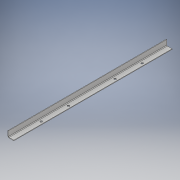
# Autodesk Inventor part: L_Profile
Saved by Autodesk Inventor 2019.3 (Build 233278000, 278)
## iProperties
Created: 2019-01-16
Part Number: L_Profile
Material: Generisch
Document SubType Name: Blech
Designer: Jonas
Density: 1 g/cm^3
Sheet Metal Rule: Standard_mm
Appearance: Vorgabe
Author: Jonas
Autodesk Inventor part; units mm, degrees
ref_plane "YZ Plane" through (0, 0, 0) normal (1, 0, 0) x (0, 1, 0)
ref_plane "XZ Plane" through (0, 0, 0) normal (0, 1, 0) x (-1, 0, 0)
ref_plane "XY Plane" through (0, 0, 0) normal (0, 0, 1) x (1, 0, 0)
sketch "Skizze3" plane through (0, 0, 0) normal (0, 1, 0) x (-1, 0, 0)
  line L0 (-5, 134) -> (5, 134)
  line L1 (5, 134) -> (5, -134)
  line L2 (5, -134) -> (-5, -134)
  line L3 (-5, -134) -> (-5, 134)
  line L4 (-5, 134) -> (5, -134) construction
  line L5 (5, 134) -> (-5, -134) construction
  point P0 (0, 0)
  dimension "d4" = 268
  dimension "d5" = 10
  measures "d4" distance of L0.end L1.end
  measures "d5" distance of L1.end L2.end
extrude "Grobblech1" add sketch "Skizze3" along normal blind 1
sketch "Skizze4" plane through (-4, 0, 134) normal (-1, 0, 0) x (0, -1, 0)
  line L0 (0, -268) -> (0, 0)
  line L1 (0, 0) -> (-10, 0)
  line L2 (-10, 0) -> (-10, -268)
  line L3 (-10, -268) -> (0, -268)
  constraints: 6 end point, 1 horizontal, 1 perpendicular, 1 vertical
edge flange "Lasche1" height 10 angle 90 thickness 1 bend radius 1 thickness toward (-1, 0, 0) relief tear relief width 1 relief depth 0.5 edges at (-5, 1, 0) wall of the first edge with corners at (-4, 0, -134) (-4, 0, 134) (-4, 10, 134) (-4, 10, -134)
bend "Biegung1"
corner "Ecke1"
sketch "Skizze5" plane through (0, 0, 0) normal (0, -1, 0) x (1, 0, 0)
  point P0 (1, 83.5)
hole "Bohrung1" at (1, 0, 83.5) direction (0, 1, 0) diameter 3.4 depth 1
sketch "Skizze6" plane through (0, 0, 0) normal (0, -1, 0) x (1, 0, 0)
  point P0 (1, 37.5)
hole "Bohrung3" at (1, 0, 37.5) direction (0, 1, 0) diameter 3.4 depth 1
sketch "Skizze7" plane through (0, 0, 0) normal (0, -1, 0) x (1, 0, 0)
  point P0 (1, -87.5)
hole "Bohrung5" at (1, 0, -87.5) direction (0, 1, 0) diameter 3.4 depth 1
sketch "Skizze8" plane through (0, 0, 0) normal (0, -1, 0) x (1, 0, 0)
  point P0 (1, -41.5)
hole "Bohrung7" at (1, 0, -41.5) direction (0, 1, 0) diameter 3.4 depth 1
equation "\"d6\" = Stärke"
equation "\"d7\" = BreiteBiegungsfreistellung"
equation "\"d8\" = TiefeBiegungsfreistellung"
equation "\"d9\" = MinimalRest"
equation "\"d10\" = Übergangsradius"
equation "\"d13\" = Biegeradius"
equation "\"d14\" = GrößeEckenfreistellung"
equation "\"d15\" = Abstandsgröße"
equation "\"d16\" = JacobiRadiusGröße"
equation "\"Biegeradius\" = Stärke"
equation "\"BreiteBiegungsfreistellung\" = Stärke"
equation "\"TiefeBiegungsfreistellung\" = 0.5 * Stärke"
equation "\"GrößeEckenfreistellung\" = 4 * Stärke"
equation "\"MinimalRest\" = 2 * Stärke"
equation "\"Übergangsradius\" = Biegeradius"
equation "\"JacobiRadiusGröße\" = Biegeradius"
equation "\"Abstandsgröße\" = Stärke"
equation "\"Stärke\" = 1"
